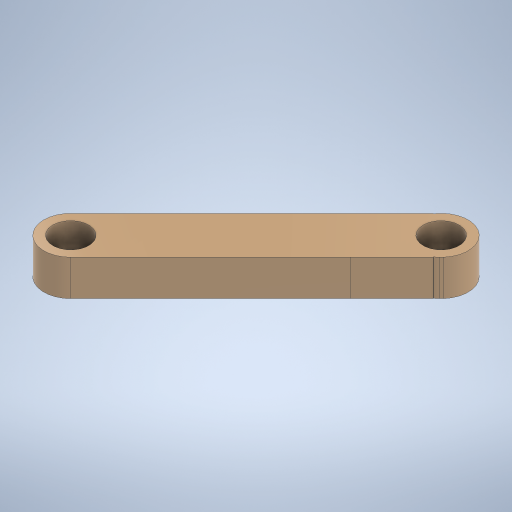
# Autodesk Inventor part: link
Saved by Autodesk Inventor 2024 (Build 280153000, 153)
## iProperties
Created: 2024-10-07
Part Number: link
Material: Generic
Document SubType Name: Modeling
Designer: m_kni
Density: 1 g/cm^3
Appearance: Default
Author: m_kni
Autodesk Inventor part; units mm, degrees
ref_plane "YZ Plane" through (0, 0, 0) normal (1, 0, 0) x (0, 1, 0)
ref_plane "XZ Plane" through (0, 0, 0) normal (0, 1, 0) x (-1, 0, 0)
ref_plane "XY Plane" through (0, 0, 0) normal (0, 0, 1) x (1, 0, 0)
sketch "Sketch1" plane through (0, 0, 0) normal (0, 1, 0) x (-1, 0, 0)
  circle A0 centre (-0.0319, -8.4999) radius 1.5
  circle A1 centre (8.4996, 0.0794) radius 1.5
  circle A2 centre (-8.4996, 0.0788) radius 1.5
  circle A3 centre (-0.0313, 8.4999) radius 1.5
  line L0 (-12.7, 12.7) -> (12.7, 12.7)
  line L1 (12.7, 12.7) -> (12.7, -12.7)
  line L2 (12.7, -12.7) -> (-12.7, -12.7)
  line L3 (-12.7, -12.7) -> (-12.7, 12.7)
  line L4 (-12.7, 12.7) -> (12.7, -12.7) construction
  line L5 (12.7, 12.7) -> (-12.7, -12.7) construction
  line L6 (-11.4771, 11.4771) -> (11.4771, 11.4771)
  line L7 (11.4771, 11.4771) -> (11.4771, -11.4771)
  line L8 (11.4771, -11.4771) -> (-11.4771, -11.4771)
  line L9 (-11.4771, -11.4771) -> (-11.4771, 11.4771)
  line L10 (-11.4771, 11.4771) -> (11.4771, -11.4771) construction
  line L11 (11.4771, 11.4771) -> (-11.4771, -11.4771) construction
  line L12 (-25.4, -25.4) -> (25.4, -25.4)
  line L13 (25.4, -25.4) -> (25.4, 25.4)
  line L14 (25.4, 25.4) -> (-25.4, 25.4)
  line L15 (-25.4, 25.4) -> (-25.4, -25.4)
  line L16 (-25.4, -25.4) -> (25.4, 25.4) construction
  line L17 (25.4, -25.4) -> (-25.4, 25.4) construction
  circle A4 centre (0, 0) radius 5.5
  circle A5 centre (11.4771, 11.4771) radius 5.5
  circle A6 centre (11.4771, -11.4771) radius 5.5
  circle A7 centre (-11.4771, 11.4771) radius 5.5
  circle A8 centre (-11.4771, -11.4771) radius 5.5
  circle A9 centre (-25.4, 25.4) radius 5.5
  circle A10 centre (25.4, 25.4) radius 5.5
  circle A11 centre (25.4, -25.4) radius 5.5
  circle A12 centre (-25.4, -25.4) radius 5.5
  line L18 (7.588, 15.3662) -> (21.5109, 29.2891)
  line L19 (29.2891, 21.5109) -> (15.3662, 7.588)
  line L20 (15.3662, -7.588) -> (29.2891, -21.5109)
  line L21 (-7.588, -15.3662) -> (-21.5109, -29.2891)
  line L22 (-29.2891, 21.5109) -> (-15.3662, 7.588)
  line L23 (7.588, -15.3662) -> (21.5109, -29.2891)
  line L24 (-15.3365, -7.5586) -> (-29.2595, -21.4815)
  line L25 (-7.6475, 15.4248) -> (-21.5108, 29.289)
  line L26 (-35, -35) -> (35, -35)
  line L27 (35, -35) -> (35, 35)
  line L28 (35, 35) -> (-35, 35)
  line L29 (-35, 35) -> (-35, -35)
  line L30 (-35, -35) -> (35, 35) construction
  line L31 (35, -35) -> (-35, 35) construction
  circle A13 centre (11.4771, 11.4771) radius 2.5
  circle A14 centre (25.4, 25.4) radius 2.5
  line L32 (27.1678, 23.6322) -> (13.2448, 9.7093)
  line L33 (23.6682, 27.203) -> (9.7093, 13.2449)
  line L34 (0, 0) -> (0, 35)
  line L35 (35, 0) -> (0, 0)
  line L36 (-27.1678, 23.6322) -> (-13.2448, 9.7093)
  circle A15 centre (-25.4, 25.4) radius 2.5
  line L37 (-23.6682, 27.203) -> (-9.7093, 13.2449)
  circle A16 centre (-11.4771, 11.4771) radius 2.5
  circle A17 centre (25.4, -25.4) radius 2.5
  line L38 (23.6682, -27.203) -> (9.7093, -13.2449)
  line L39 (27.1678, -23.6322) -> (13.2448, -9.7093)
  circle A18 centre (11.4771, -11.4771) radius 2.5
  circle A19 centre (-11.4771, -11.4771) radius 2.5
  line L40 (-23.6682, -27.203) -> (-9.7093, -13.2449)
  line L41 (-27.1678, -23.6322) -> (-13.2448, -9.7093)
  line L42 (25.4, 25.4) -> (-25.4, -25.4) construction
  circle A20 centre (-25.4, -25.4) radius 2.5
  circle A21 centre (0, 0) radius 8.509
  circle A22 centre (-6.0168, -6.0168) radius 1.5
  line L43 (-25.4, -25.4) -> (-17.6218, -17.6218)
  circle A23 centre (-17.6218, -17.6218) radius 5.5
  circle A24 centre (-6.0168, -6.0168) radius 2.25
  line L44 (-16.1218, -19.2989) -> (-4.5109, -7.6886)
  line L45 (-19.2988, -16.1217) -> (-7.6081, -4.4261)
  circle A25 centre (-21.5109, -21.5109) radius 1.5
  circle A26 centre (-21.5109, -21.5109) radius 2.25
  line L46 (-19.2988, -16.1217) -> (-23.1879, -20.0108)
  line L47 (-16.1218, -19.2989) -> (-19.9189, -23.1009)
  point P0 (-22.7602, -19.5832)
  point P1 (-22.7428, -19.6281)
  point P2 (-23.011, -19.8339)
  point P3 (-19.6281, -22.7428)
  point P4 (-19.5799, -22.7615)
  dimension "d24" = 17.018
  dimension "d0" = 8.5
  dimension "d1" = 8.5
  dimension "d2" = 8.5
  dimension "d3" = 8.5
  dimension "d4" = 3
  dimension "d5" = 3
  dimension "d6" = 3
  dimension "d7" = 3
  dimension "d8" = 25.4
  dimension "d9" = 25.4
  dimension "d10" = 50.8
  dimension "d11" = 50.8
  dimension "d12" = 11
  dimension "d13" = 11
  dimension "d14" = 11
  dimension "d15" = 11
  dimension "d16" = 11
  dimension "d17" = 11
  dimension "d18" = 11
  dimension "d19" = 11
  dimension "d20" = 11
  dimension "d21" = 70
  dimension "d22" = 5
  dimension "d23" = 5
  dimension "d25" = 3
  dimension "d26" = 11
  dimension "d28" = 4.5
  dimension "d33" = 3
  dimension "d34" = 4.5
  constraints: 96 end point, 36 point on circle, 25 centre point, 22 coincident, 18 symmetric about line, 15 tangent, 11 midpoint, 10 parallel, 5 horizontal, 5 perpendicular, 5 point on line, 13 other
  measures "d0" distance of point (-0.032, -8.5) point (0, 0)
  measures "d1" distance of point (-8.5, 0.079) point (0, 0)
  measures "d2" distance of point (-0.031, 8.5) point (0, 0)
  measures "d3" distance of point (8.5, 0.079) point (0, 0)
  measures "d4" diameter of A0
  measures "d5" diameter of A1
  measures "d6" diameter of A2
  measures "d7" diameter of A3
  measures "d8" distance of L1.end L2.end
  measures "d9" distance of L0.end L1.end
  measures "d10" distance of L14.end L13.end
  measures "d11" distance of L13.end L12.end
  measures "d12" diameter of A4
  measures "d13" diameter of A5
  measures "d14" diameter of A6
  measures "d15" diameter of A7
  measures "d16" diameter of A8
  measures "d17" diameter of A9
  measures "d18" diameter of A10
  measures "d19" diameter of A11
  measures "d20" diameter of A12
  measures "d21" distance of L28.end L27.end
  measures "d22" diameter of A13
  measures "d23" diameter of A14
  measures "d25" diameter of A22
  measures "d26" distance of L43.start L43.end
  measures "d28" diameter of A24
  measures "d33" diameter of A25
  measures "d34" diameter of A26
extrude "Extrusion1" add sketch "Sketch1" along normal blind 3 contours A24 A8 A21 A22 | A21 A22 A24 | L44 A8 A24 | A24 A8 | A8 L44 L8 A19 L9 L45 A24 | A8 L45 A24 | L44 A19 L8 | A19 L44 L2 L3 L45 L9 L8 | L8 L9 A19 | L9 A19 L45 | L44 A19 L45 L3 L2 | L44 A23 L45 A19 | L44 A8 L45 A23 | L44 L47 A23 A26 L46 L45 A8 | A26 L43 A25 A12 | A12 A25 A23 A26 | A23 A25 L43 A26 | A26 A12 A25 L43 | A26 A23 A25 A12 | A26 L43 A25 A23
body "Solid1"
